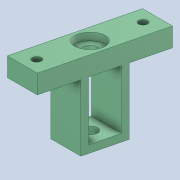
# Autodesk Inventor part: Part2
Saved by Autodesk Inventor 2020 (Build 240168000, 168)
## iProperties
Created: 2019-05-14
Part Number: Part2
Material: ABS Plastic
Document SubType Name: Modeling
Designer: kimhos
Density: 1.06 g/cm^3
Appearance: Smooth - Dark Sea Green
Author: kimhos
Autodesk Inventor part; units mm, degrees
ref_plane "YZ Plane" through (0, 0, 0) normal (1, 0, 0) x (0, 1, 0)
ref_plane "XZ Plane" through (0, 0, 0) normal (0, 1, 0) x (-1, 0, 0)
ref_plane "XY Plane" through (0, 0, 0) normal (0, 0, 1) x (1, 0, 0)
sketch "Sketch1" plane through (0, 0, 0) normal (0, 0, 1) x (1, 0, 0)
  line L0 (-7.0076, 0.0013) -> (-0.0076, 0.0013)
  line L1 (-7.0076, -1.9987) -> (-2.5076, -1.9987)
  line L2 (-2.5076, -1.9987) -> (-2.5076, -8.9987)
  line L3 (-2.5076, -8.9987) -> (-0.0076, -8.9987)
  line L4 (-7.0076, 0.0013) -> (-7.0076, -1.9987)
  line L5 (6.9924, 0.0013) -> (-0.0076, 0.0013)
  line L6 (6.9924, -1.9987) -> (2.4924, -1.9987)
  line L7 (2.4924, -1.9987) -> (2.4924, -8.9987)
  line L8 (2.4924, -8.9987) -> (-0.0076, -8.9987)
  line L9 (6.9924, 0.0013) -> (6.9924, -1.9987)
  line L10 (-2.5076, -7.0289) -> (-1.7076, -7.0289)
  line L11 (2.4924, -7.0289) -> (1.6924, -7.0289)
  line L12 (-0.0076, -8.9987) -> (-0.0076, -8.1987)
  point P0 (0, 0)
  point P1 (8.0042, -1.0097)
  point P2 (8.0042, -1.0097)
  dimension "d0" = 7
  dimension "d4" = 7
  dimension "d5" = 2
  dimension "d8" = 2.5
  dimension "d9" = 4.5
  dimension "d49" = 2.5
  dimension "d114" = 0.8
  dimension "d117" = 0.8
  dimension "d118" = 0.8
  constraints: 26 end point, 4 horizontal, 3 equal length, 2 point on line, 2 vertical, 1 coincident, 1 perpendicular, 2 other
  measures "d0" distance of L0.start L0.end
  measures "d4" distance of L1.end L2.end
  measures "d5" distance of L0.start L1.start
  measures "d8" distance of L2.end L3.end
  measures "d9" distance of L1.start L1.end
  measures "d49" distance of L7.end L3.end
  measures "d114" distance of L10.start L10.end
  measures "d117" distance of L11.start L11.end
  measures "d118" distance of L3.end L12.end
extrude "Extrusion1" add sketch "Sketch1" along normal mid plane 4
shell "Shell1" thickness 0.8 removed faces 1 at (0.8258, -6.6653, 2)
move faces "Move1" translate (0, -1.2, 0) faces at (2.0591, -0.7987, -0.1333)
move faces "Move2" translate (0, 0, -1) faces at (-0.5742, -6.132, -1.2)
sketch "Sketch16" plane through (-2.5076, -8.9987, 2) normal (0, -1, 0) x (1, 0, 0)
  circle A0 centre (2.5076, -2) radius 0.8
  line L0 (5, -4) -> (5, 0) projected
  line L1 (5, -2) -> (2.5076, -2)
  line L2 (2.5076, -2) -> (5.0076, -2)
  dimension "d51" = 1.6
  dimension "d102" = 2.5
  constraints: 4 end point, 1 centre point, 1 coincident, 1 horizontal, 1 midpoint, 1 point on line
  measures "d51" diameter of A0
  measures "d102" distance of L1.end L2.end
hole "Hole4" at (0, -8.9987, 0) direction (0, 1, 0) diameter 1.6 depth 2
sketch "Sketch18" plane through (-7.0076, 0.0013, 2) normal (0, 1, 0) x (1, 0, 0)
  line L0 (14, 4) -> (14, 0) projected
  line L1 (14, 2) -> (12.5, 2)
  circle A0 centre (12.5, 2) radius 0.5
  point P0 (7.0076, 2)
  dimension "d67" = 1.5
  dimension "d68" = 1
  constraints: 2 end point, 1 centre point, 1 coincident, 1 horizontal, 1 midpoint
  measures "d67" distance of L1.start L1.end
  measures "d68" diameter of A0
hole "Hole6" at (5.4924, 0.0013, 0) direction (0, -1, 0) diameter 1 depth 4
sketch "Sketch19" plane through (-7.0076, 0.0013, 2) normal (0, 1, 0) x (1, 0, 0)
  line L0 (0, 4) -> (0, 0) projected
  line L1 (0, 2) -> (1.5, 2)
  circle A0 centre (1.5, 2) radius 0.5
  point P0 (7.0076, 2)
  dimension "d76" = 1.5
  dimension "d77" = 1
  constraints: 2 end point, 1 centre point, 1 coincident, 1 horizontal, 1 midpoint
  measures "d76" distance of L1.start L1.end
  measures "d77" diameter of A0
hole "Hole7" at (-5.5076, 0.0013, 0) direction (0, -1, 0) diameter 1 depth 4
sketch "Sketch21" plane through (-7.0076, 0.0013, 2) normal (0, 1, 0) x (1, 0, 0)
  line L0 (0, 4) -> (0, 0) projected
  line L1 (0, 2) -> (7, 2)
  line L2 (7, 2) -> (7, 4)
  line L3 (7, 4) -> (7, 2)
  circle A0 centre (7, 2) radius 1.5
  point P0 (6.0076, 2)
  dimension "d103" = 7
  dimension "d104" = 2
  dimension "d105" = 3
  constraints: 6 end point, 1 centre point, 1 coincident, 1 collinear, 1 horizontal, 1 midpoint, 1 vertical
  measures "d103" distance of L1.start L1.end
  measures "d104" distance of L2.end L1.end
  measures "d105" diameter of A0
hole "Hole9" at (-0.0076, 0.0013, 0) direction (0, -1, 0) diameter 1.6 depth 4.8 counterbore diameter 3.2 counterbore depth 0.8
body "Solid1"
